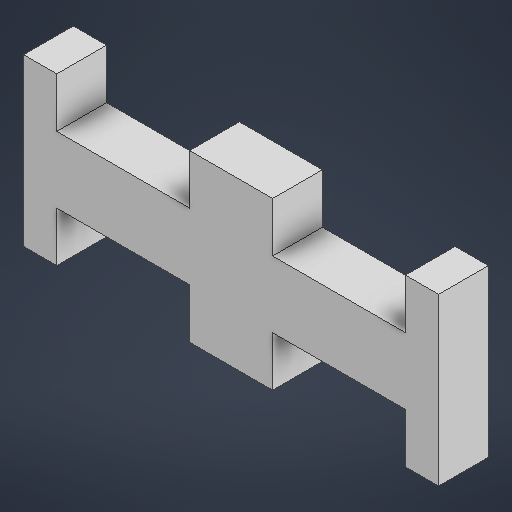
# Autodesk Inventor part: techoProctetorSensorHal
Saved by Autodesk Inventor 2026 (Build 300175000, 175)
## iProperties
Created: 2026-05-15
Part Number: techoProctetorSensorHal
Material: Generic
Document SubType Name: Modeling
Designer: juana
Density: 1 g/cm^3
Appearance: Default
Author: juana
Autodesk Inventor part; units mm, degrees
ref_plane "YZ Plane" through (0, 0, 0) normal (1, 0, 0) x (0, 1, 0)
ref_plane "XZ Plane" through (0, 0, 0) normal (0, 1, 0) x (-1, 0, 0)
ref_plane "XY Plane" through (0, 0, 0) normal (0, 0, 1) x (1, 0, 0)
sketch "Sketch1" plane through (0, 0, 0) normal (0, 0, 1) x (1, 0, 0)
  line L0 (0, 10.2918) -> (25, 10.2918)
  line L1 (25, 10.2918) -> (25, 0.2918)
  line L2 (25, 0.2918) -> (0, 0.2918)
  line L3 (0, 0.2918) -> (0, 10.2918)
  line L4 (2, 0.2918) -> (10, 0.2918)
  line L5 (10, 0.2918) -> (10, 3.2918)
  line L6 (10, 3.2918) -> (2, 3.2918)
  line L7 (2, 3.2918) -> (2, 0.2918)
  line L8 (0, 5.2918) -> (25, 5.2918) construction
  line L9 (12.5, 10.2918) -> (12.5, 0.2918) construction
  line L10 (23, 0.2918) -> (15, 0.2918)
  line L11 (15, 0.2918) -> (15, 3.2918)
  line L12 (15, 3.2918) -> (23, 3.2918)
  line L13 (23, 3.2918) -> (23, 0.2918)
  line L14 (2, 10.2918) -> (10, 10.2918)
  line L15 (10, 10.2918) -> (10, 7.2918)
  line L16 (10, 7.2918) -> (2, 7.2918)
  line L17 (2, 7.2918) -> (2, 10.2918)
  line L18 (23, 10.2918) -> (15, 10.2918)
  line L19 (15, 10.2918) -> (15, 7.2918)
  line L20 (15, 7.2918) -> (23, 7.2918)
  line L21 (23, 7.2918) -> (23, 10.2918)
  point P0 (0, 0)
  dimension "d0" = 25
  dimension "d1" = 10
  dimension "d2" = 3
  dimension "d3" = 2
  dimension "d4" = 8
  constraints: 44 end point, 12 symmetric about line, 4 midpoint, 4 parallel, 2 horizontal, 2 perpendicular, 1 point on line
  measures "d0" distance of L0.start L0.end
  measures "d1" distance of L0.end L1.end
  measures "d2" distance of L6.end L4.start
  measures "d3" distance between parallel lines of L3 L7
  measures "d4" distance of L5.end L6.end
extrude "Extrusion1" add sketch "Sketch1" along normal blind 3 contours L0 L17 L16 L15 L19 L20 L21 L1 L2 L13 L12 L11 L5 L6 L7 L3
body "Solid1"
